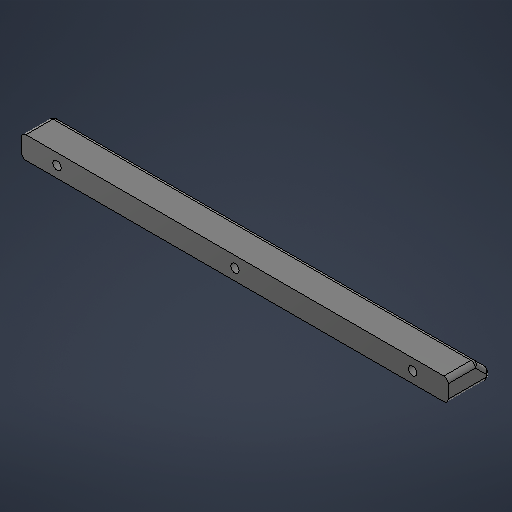
# Autodesk Inventor part: 3DPRINT,BELT,GUARD
Saved by Autodesk Inventor 2026.1 (Build 301233020, 233B)
## iProperties
Created: 2026-04-01
Part Number: 3DPRINT,BELT,GUARD
Material: ABS Plastic
Document SubType Name: Modeling
Designer: Owen L
Mass: 68.0389 g
Surface Area: 270.876 cm^2
Volume: 130.153 cm^3
Density: 0.522761 g/cm^3
Appearance: Smooth - Black
Author: Owen L
Autodesk Inventor part; units mm, degrees
ref_plane "YZ Plane" through (0, 0, 0) normal (1, 0, 0) x (0, 1, 0)
ref_plane "XZ Plane" through (0, 0, 0) normal (0, 1, 0) x (-1, 0, 0)
ref_plane "XY Plane" through (0, 0, 0) normal (0, 0, 1) x (1, 0, 0)
sketch "Sketch1" plane through (0, 0, 0) normal (1, 0, 0) x (0, 1, 0)
  line L0 (0, 0) -> (30.1625, 0)
  line L1 (30.1625, 0) -> (30.1625, -6.35)
  line L2 (30.1625, -6.35) -> (6.35, -30.1625)
  line L3 (6.35, -30.1625) -> (0, -30.1625)
  line L4 (0, -30.1625) -> (0, 0)
  line L5 (15.875, 0) -> (15.875, -20.6375)
  point P0 (15.0812, 0)
  dimension "d0" = 30.1625
  dimension "d1" = 6.35
  dimension "d16" = 15.875
  constraints: 12 end point, 4 perpendicular, 2 point on line, 1 horizontal, 1 midpoint, 1 parallel, 1 vertical
  measures "d0" distance of L3.end L0.start
  measures "d1" distance of L2.end L3.end
  measures "d16" distance between parallel lines of L4 L5
extrude "Extrusion1" add sketch "Sketch1" along normal blind 304.8 contours L0 L5 L2 L3 L4
sketch "Sketch2" plane through (0, 0, 0) normal (0, 0, 1) x (1, 0, 0)
  line L0 (0, 15.875) -> (0, 0) projected
  line L1 (0, 0) -> (304.8, 0) projected
  point P0 (25.4, 7.9375)
  point P1 (152.4, 7.9375)
  point P2 (279.4, 7.9375)
  point P3 (152.4, 0)
  dimension "d4" = 25.4
  dimension "d5" = 7.9375
  dimension "d6" = 25.4
  constraints: 2 horizontal alignment, 1 midpoint, 1 vertical alignment
  measures "d4" distance from line of L0 point (25.4, 7.938)
  measures "d5" distance from line of L1 point (25.4, 7.938)
  measures "d6" horizontal distance of L1.end point (279.4, 7.938)
hole "Hole1" at (25.4, 7.9375, 0) at (152.4, 7.9375, 0) at (279.4, 7.9375, 0) direction (0, 0, -1) diameter 6.096 depth 9.525 tip angle 118
fillet "Fillet1" radius 3.175 11 edges at (152.4, 6.35, -30.1625) (152.4, 0, -30.1625) (0, 11.1125, -25.4) (0, 3.175, -30.1625) (0, 0, -15.0812) (304.8, 3.175, -30.1625) (304.8, 0, -15.0812) (304.8, 11.1125, -25.4) (152.4, 15.875, -20.6375) (304.8, 15.875, -10.3188) (0, 15.875, -10.3188)
body "Solid1"
